Autodesk Fusion 360 part; units mm, degrees
note: some values were not read from the file. Set by a fixed rule: the direction of a hole.
(part 2 of 6)
sketch "Sketch2" plane through (0, 0, 2) normal (0, 0, 1) x (-1, 0, 0)
  line L0 (-25, -25) -> (-154, -25)
  line L1 (-154, -25) -> (-154, -111)
  line L2 (-154, -111) -> (-25, -111)
  line L3 (-25, -111) -> (-25, -25)
  spline S0 degree 3 poles (-57.3506, -87.5946) (-57.8745, -87.5946) (-58.3983, -87.5946) (-58.9381, -87.5946) knots 0 0 0 0 1 1 1 1
  spline S1 degree 3 poles (-58.9381, -87.5946) (-58.9624, -85.5487) (-58.8869, -83.5156) (-58.7793, -81.4728) knots 0 0 0 0 1 1 1 1
  spline S2 degree 3 poles (-58.7793, -81.4728) (-58.764, -81.1715) (-58.7487, -80.8702) (-58.7335, -80.5689) knots 0 0 0 0 1 1 1 1
  spline S3 degree 3 poles (-58.7335, -80.5689) (-58.6965, -79.8416) (-58.6588, -79.1143) (-58.6206, -78.3871) knots 0 0 0 0 1 1 1 1
  spline S4 degree 3 poles (-58.6206, -78.3871) (-58.3587, -78.3871) (-58.0967, -78.3871) (-57.8268, -78.3871) knots 0 0 0 0 1 1 1 1
  spline S5 degree 3 poles (-57.8268, -78.3871) (-57.6309, -79.1758) (-57.6136, -79.9701) (-57.5788, -80.7782) knots 0 0 0 0 1 1 1 1
  spline S6 degree 3 poles (-57.5788, -80.7782) (-57.5721, -80.9263) (-57.5653, -81.0744) (-57.5584, -81.227) knots 0 0 0 0 1 1 1 1
  spline S7 degree 3 poles (-57.5584, -81.227) (-57.5124, -82.2924) (-57.4938, -83.3532) (-57.5093, -84.4196) knots 0 0 0 0 1 1 1 1
  spline S8 degree 3 poles (-57.5093, -84.4196) (-55.2128, -84.0888) (-53.0605, -83.6004) (-50.8806, -82.8013) knots 0 0 0 0 1 1 1 1
  spline S9 degree 3 poles (-50.8806, -82.8013) (-50.4467, -82.6454) (-50.0096, -82.5004) (-49.5718, -82.3558) knots 0 0 0 0 1 1 1 1
  spline S10 degree 3 poles (-49.5718, -82.3558) (-51.0894, -79.4889) (-52.6118, -76.6254) (-54.1756, -73.7833) knots 0 0 0 0 1 1 1 1
  spline S11 degree 3 poles (-54.1756, -73.7833) (-54.0184, -73.6262) (-53.8613, -73.469) (-53.6993, -73.3071) knots 0 0 0 0 1 1 1 1
  spline S12 degree 3 poles (-53.6993, -73.3071) (-53.1237, -73.4989) (-53.084, -73.6261) (-52.7921, -74.1393) knots 0 0 0 0 1 1 1 1
  spline S13 degree 3 poles (-52.7921, -74.1393) (-52.6693, -74.3518) (-52.6693, -74.3518) (-52.5441, -74.5686) knots 0 0 0 0 1 1 1 1
  spline S14 degree 3 poles (-52.5441, -74.5686) (-52.4571, -74.722) (-52.3701, -74.8754) (-52.2805, -75.0335) knots 0 0 0 0 1 1 1 1
  spline S15 degree 3 poles (-52.2805, -75.0335) (-52.0957, -75.353) (-51.9105, -75.6724) (-51.7249, -75.9916) knots 0 0 0 0 1 1 1 1
  spline S16 degree 3 poles (-51.7249, -75.9916) (-51.631, -76.1532) (-51.537, -76.3149) (-51.4403, -76.4815) knots 0 0 0 0 1 1 1 1
  spline S17 degree 3 poles (-51.4403, -76.4815) (-51.0199, -77.195) (-50.5812, -77.8963) (-50.1374, -78.5954) knots 0 0 0 0 1 1 1 1
  spline S18 degree 3 poles (-50.1374, -78.5954) (-50.0252, -78.7727) (-50.0252, -78.7727) (-49.9108, -78.9535) knots 0 0 0 0 1 1 1 1
  spline S19 degree 3 poles (-49.9108, -78.9535) (-49.3861, -79.7779) (-48.8466, -80.592) (-48.3018, -81.4033) knots 0 0 0 0 1 1 1 1
  spline S20 degree 3 poles (-48.3018, -81.4033) (-47.1239, -80.6157) (-46.0109, -79.8094) (-45.0078, -78.8038) knots 0 0 0 0 1 1 1 1
  spline S21 degree 3 poles (-45.0078, -78.8038) (-44.9283, -78.7245) (-44.8489, -78.6453) (-44.767, -78.5636) knots 0 0 0 0 1 1 1 1
  spline S22 degree 3 poles (-44.767, -78.5636) (-44.3785, -78.1633) (-44.0684, -77.795) (-43.8568, -77.2758) knots 0 0 0 0 1 1 1 1
  spline S23 degree 3 poles (-43.8568, -77.2758) (-45.1932, -76.2876) (-46.5379, -75.3133) (-47.8979, -74.3579) knots 0 0 0 0 1 1 1 1
  spline S24 degree 3 poles (-47.8979, -74.3579) (-48.8336, -73.6998) (-49.7613, -73.031) (-50.686, -72.3575) knots 0 0 0 0 1 1 1 1
  spline S25 degree 3 poles (-50.686, -72.3575) (-51.3445, -71.8797) (-52.0085, -71.4118) (-52.6805, -70.9531) knots 0 0 0 0 1 1 1 1
  spline S26 degree 3 poles (-52.6805, -70.9531) (-52.8271, -70.8525) (-52.9738, -70.7519) (-53.1249, -70.6482) knots 0 0 0 0 1 1 1 1
  spline S27 degree 3 poles (-53.1249, -70.6482) (-53.4109, -70.4526) (-53.6978, -70.2583) (-53.9857, -70.0655) knots 0 0 0 0 1 1 1 1
  spline S28 degree 3 poles (-53.9857, -70.0655) (-54.1143, -69.9774) (-54.2428, -69.8892) (-54.3753, -69.7984) knots 0 0 0 0 1 1 1 1
  spline S29 degree 3 poles (-54.3753, -69.7984) (-54.5475, -69.6822) (-54.5475, -69.6822) (-54.7232, -69.5636) knots 0 0 0 0 1 1 1 1
  spline S30 degree 3 poles (-54.7232, -69.5636) (-54.8044, -69.4893) (-54.8857, -69.4149) (-54.9693, -69.3383) knots 0 0 0 0 1 1 1 1
  spline S31 degree 3 poles (-54.9693, -69.3383) (-54.9693, -68.8621) (-54.9693, -68.8621) (-54.8106, -68.5446) knots 0 0 0 0 1 1 1 1
  spline S32 degree 3 poles (-54.8106, -68.5446) (-54.2842, -68.6454) (-53.922, -68.8386) (-53.4767, -69.1337) knots 0 0 0 0 1 1 1 1
  spline S33 degree 3 poles (-53.4767, -69.1337) (-53.3377, -69.2251) (-53.1987, -69.3165) (-53.0555, -69.4107) knots 0 0 0 0 1 1 1 1
  spline S34 degree 3 poles (-53.0555, -69.4107) (-52.829, -69.5615) (-52.829, -69.5615) (-52.598, -69.7153) knots 0 0 0 0 1 1 1 1
  spline S35 degree 3 poles (-52.598, -69.7153) (-52.2685, -69.9326) (-51.939, -70.1499) (-51.6095, -70.3671) knots 0 0 0 0 1 1 1 1
  spline S36 degree 3 poles (-51.6095, -70.3671) (-51.4323, -70.4844) (-51.2551, -70.6016) (-51.0779, -70.7189) knots 0 0 0 0 1 1 1 1
  spline S37 degree 3 poles (-51.0779, -70.7189) (-50.5065, -71.0968) (-49.9333, -71.472) (-49.3598, -71.8467) knots 0 0 0 0 1 1 1 1
  spline S38 degree 3 poles (-49.3598, -71.8467) (-49.162, -71.9759) (-48.9642, -72.1052) (-48.7665, -72.2345) knots 0 0 0 0 1 1 1 1
  spline S39 degree 3 poles (-48.7665, -72.2345) (-48.6684, -72.2985) (-48.5704, -72.3626) (-48.4694, -72.4286) knots 0 0 0 0 1 1 1 1
  spline S40 degree 3 poles (-48.4694, -72.4286) (-46.1202, -73.9643) (-46.1202, -73.9643) (-45.0041, -74.716) knots 0 0 0 0 1 1 1 1
  spline S41 degree 3 poles (-45.0041, -74.716) (-44.8702, -74.8061) (-44.7363, -74.8962) (-44.5984, -74.989) knots 0 0 0 0 1 1 1 1
  spline S42 degree 3 poles (-44.5984, -74.989) (-44.356, -75.1526) (-44.1141, -75.3169) (-43.8728, -75.4819) knots 0 0 0 0 1 1 1 1
  spline S43 degree 3 poles (-43.8728, -75.4819) (-43.3554, -75.8717) (-43.3554, -75.8717) (-42.7456, -76.0058) knots 0 0 0 0 1 1 1 1
  spline S44 degree 3 poles (-42.7456, -76.0058) (-42.2217, -75.0105) (-41.6978, -74.0151) (-41.1581, -72.9896) knots 0 0 0 0 1 1 1 1
  spline S45 degree 3 poles (-41.1581, -72.9896) (-41.6296, -72.8324) (-42.1011, -72.6752) (-42.5868, -72.5133) knots 0 0 0 0 1 1 1 1
  spline S46 degree 3 poles (-42.5868, -72.5133) (-42.8781, -72.3992) (-43.168, -72.2814) (-43.4555, -72.1583) knots 0 0 0 0 1 1 1 1
  spline S47 degree 3 poles (-43.4555, -72.1583) (-43.6096, -72.0926) (-43.7637, -72.0269) (-43.9225, -71.9592) knots 0 0 0 0 1 1 1 1
  spline S48 degree 3 poles (-43.9225, -71.9592) (-44.1644, -71.855) (-44.1644, -71.855) (-44.4112, -71.7487) knots 0 0 0 0 1 1 1 1
  spline S49 degree 3 poles (-44.4112, -71.7487) (-44.5807, -71.6761) (-44.7502, -71.6036) (-44.9249, -71.5288) knots 0 0 0 0 1 1 1 1
  spline S50 degree 3 poles (-44.9249, -71.5288) (-45.2807, -71.3763) (-45.6363, -71.2235) (-45.9919, -71.0705) knots 0 0 0 0 1 1 1 1
  spline S51 degree 3 poles (-45.9919, -71.0705) (-46.5371, -70.836) (-47.0827, -70.6025) (-47.6284, -70.3693) knots 0 0 0 0 1 1 1 1
  spline S52 degree 3 poles (-47.6284, -70.3693) (-47.9749, -70.2206) (-48.3213, -70.0719) (-48.6677, -69.9231) knots 0 0 0 0 1 1 1 1
  spline S53 degree 3 poles (-48.6677, -69.9231) (-48.8309, -69.8533) (-48.9941, -69.7835) (-49.1623, -69.7116) knots 0 0 0 0 1 1 1 1
  spline S54 degree 3 poles (-49.1623, -69.7116) (-49.3134, -69.6464) (-49.4645, -69.5812) (-49.6201, -69.5141) knots 0 0 0 0 1 1 1 1
  spline S55 degree 3 poles (-49.6201, -69.5141) (-49.753, -69.457) (-49.8858, -69.3999) (-50.0226, -69.3411) knots 0 0 0 0 1 1 1 1
  spline S56 degree 3 poles (-50.0226, -69.3411) (-50.3656, -69.1796) (-50.3656, -69.1796) (-50.8418, -68.8621) knots 0 0 0 0 1 1 1 1
  spline S57 degree 3 poles (-50.8418, -68.8621) (-50.7633, -68.5477) (-50.7633, -68.5477) (-50.6831, -68.2271) knots 0 0 0 0 1 1 1 1
  spline S58 degree 3 poles (-50.6831, -68.2271) (-49.5395, -68.587) (-48.4525, -69.0329) (-47.3549, -69.5138) knots 0 0 0 0 1 1 1 1
  spline S59 degree 3 poles (-47.3549, -69.5138) (-47.178, -69.5907) (-47.0011, -69.6675) (-46.8188, -69.7467) knots 0 0 0 0 1 1 1 1
  spline S60 degree 3 poles (-46.8188, -69.7467) (-46.2578, -69.9903) (-45.6973, -70.2347) (-45.1368, -70.4793) knots 0 0 0 0 1 1 1 1
  spline S61 degree 3 poles (-45.1368, -70.4793) (-44.3948, -70.8031) (-43.6524, -71.126) (-42.9099, -71.4486) knots 0 0 0 0 1 1 1 1
  spline S62 degree 3 poles (-42.9099, -71.4486) (-42.7389, -71.5235) (-42.568, -71.5984) (-42.3918, -71.6755) knots 0 0 0 0 1 1 1 1
  spline S63 degree 3 poles (-42.3918, -71.6755) (-42.2344, -71.7439) (-42.0769, -71.8123) (-41.9147, -71.8828) knots 0 0 0 0 1 1 1 1
  spline S64 degree 3 poles (-41.9147, -71.8828) (-41.7759, -71.9434) (-41.637, -72.004) (-41.494, -72.0664) knots 0 0 0 0 1 1 1 1
  spline S65 degree 3 poles (-41.494, -72.0664) (-41.1687, -72.2148) (-41.1687, -72.2148) (-40.8406, -72.1958) knots 0 0 0 0 1 1 1 1
  spline S66 degree 3 poles (-40.8406, -72.1958) (-40.5787, -71.3576) (-40.3167, -70.5194) (-40.0468, -69.6558) knots 0 0 0 0 1 1 1 1
  spline S67 degree 3 poles (-40.0468, -69.6558) (-40.425, -69.5969) (-40.425, -69.5969) (-40.8108, -69.5368) knots 0 0 0 0 1 1 1 1
  spline S68 degree 3 poles (-40.8108, -69.5368) (-41.7318, -69.3834) (-42.6454, -69.2019) (-43.5592, -69.0109) knots 0 0 0 0 1 1 1 1
  spline S69 degree 3 poles (-43.5592, -69.0109) (-43.7596, -68.9694) (-43.7596, -68.9694) (-43.964, -68.927) knots 0 0 0 0 1 1 1 1
  spline S70 degree 3 poles (-43.964, -68.927) (-44.0895, -68.9005) (-44.215, -68.8739) (-44.3443, -68.8466) knots 0 0 0 0 1 1 1 1
  spline S71 degree 3 poles (-44.3443, -68.8466) (-44.4568, -68.8228) (-44.5694, -68.7991) (-44.6854, -68.7746) knots 0 0 0 0 1 1 1 1
  spline S72 degree 3 poles (-44.6854, -68.7746) (-44.9681, -68.7033) (-44.9681, -68.7033) (-45.2856, -68.5446) knots 0 0 0 0 1 1 1 1
  spline S73 degree 3 poles (-45.2856, -68.5446) (-45.2332, -68.2826) (-45.1808, -68.0207) (-45.1268, -67.7508) knots 0 0 0 0 1 1 1 1
  spline S74 degree 3 poles (-45.1268, -67.7508) (-44.4572, -67.8377) (-43.7877, -67.9253) (-43.1182, -68.0134) knots 0 0 0 0 1 1 1 1
  spline S75 degree 3 poles (-43.1182, -68.0134) (-42.8905, -68.0433) (-42.6628, -68.073) (-42.435, -68.1025) knots 0 0 0 0 1 1 1 1
  spline S76 degree 3 poles (-42.435, -68.1025) (-42.1075, -68.1451) (-41.7801, -68.1882) (-41.4526, -68.2314) knots 0 0 0 0 1 1 1 1
  spline S77 degree 3 poles (-41.4526, -68.2314) (-41.1571, -68.2701) (-41.1571, -68.2701) (-40.8556, -68.3095) knots 0 0 0 0 1 1 1 1
  spline S78 degree 3 poles (-40.8556, -68.3095) (-40.3643, -68.3858) (-40.3643, -68.3858) (-39.8881, -68.5446) knots 0 0 0 0 1 1 1 1
  spline S79 degree 3 poles (-39.8881, -68.5446) (-39.8357, -67.7588) (-39.7833, -66.9729) (-39.7293, -66.1633) knots 0 0 0 0 1 1 1 1
  spline S80 degree 3 poles (-39.7293, -66.1633) (-40.9343, -66.1633) (-42.1392, -66.1633) (-43.3806, -66.1633) knots 0 0 0 0 1 1 1 1
  spline S81 degree 3 poles (-43.3806, -66.1633) (-43.3806, -65.9538) (-43.3806, -65.7442) (-43.3806, -65.5283) knots 0 0 0 0 1 1 1 1
  spline S82 degree 3 poles (-43.3806, -65.5283) (-41.9137, -65.5283) (-40.4469, -65.5283) (-38.9356, -65.5283) knots 0 0 0 0 1 1 1 1
  spline S83 degree 3 poles (-38.9356, -65.5283) (-38.9356, -66.6399) (-38.9521, -67.6188) (-39.0943, -68.7033) knots 0 0 0 0 1 1 1 1
  spline S84 degree 3 poles (-39.0943, -68.7033) (-38.9726, -68.711) (-38.8509, -68.7186) (-38.7256, -68.7265) knots 0 0 0 0 1 1 1 1
  spline S85 degree 3 poles (-38.7256, -68.7265) (-37.3659, -68.8206) (-36.0268, -68.9891) (-34.6791, -69.1895) knots 0 0 0 0 1 1 1 1
  spline S86 degree 3 poles (-34.6791, -69.1895) (-34.4764, -69.2191) (-34.2737, -69.2486) (-34.0649, -69.2791) knots 0 0 0 0 1 1 1 1
  spline S87 degree 3 poles (-34.0649, -69.2791) (-33.5717, -69.3511) (-33.0786, -69.4238) (-32.5856, -69.4971) knots 0 0 0 0 1 1 1 1
  spline S88 degree 3 poles (-32.5856, -69.4971) (-32.638, -70.0733) (-32.6904, -70.6496) (-32.7443, -71.2433) knots 0 0 0 0 1 1 1 1
  spline S89 degree 3 poles (-32.7443, -71.2433) (-33.6174, -71.0657) (-34.4904, -70.8878) (-35.3634, -70.7094) knots 0 0 0 0 1 1 1 1
  spline S90 degree 3 poles (-35.3634, -70.7094) (-35.6604, -70.6488) (-35.9574, -70.5883) (-36.2545, -70.5279) knots 0 0 0 0 1 1 1 1
  spline S91 degree 3 poles (-36.2545, -70.5279) (-36.6813, -70.4411) (-37.108, -70.3539) (-37.5347, -70.2666) knots 0 0 0 0 1 1 1 1
  spline S92 degree 3 poles (-37.5347, -70.2666) (-37.6677, -70.2397) (-37.8007, -70.2127) (-37.9377, -70.1849) knots 0 0 0 0 1 1 1 1
  spline S93 degree 3 poles (-37.9377, -70.1849) (-38.0616, -70.1595) (-38.1855, -70.1341) (-38.3132, -70.1079) knots 0 0 0 0 1 1 1 1
  spline S94 degree 3 poles (-38.3132, -70.1079) (-38.4221, -70.0857) (-38.531, -70.0635) (-38.6433, -70.0406) knots 0 0 0 0 1 1 1 1
  spline S95 degree 3 poles (-38.6433, -70.0406) (-38.9356, -69.9733) (-38.9356, -69.9733) (-39.4118, -69.8146) knots 0 0 0 0 1 1 1 1
  spline S96 degree 3 poles (-39.4118, -69.8146) (-39.428, -69.9942) (-39.4442, -70.1739) (-39.4608, -70.359) knots 0 0 0 0 1 1 1 1
  spline S97 degree 3 poles (-39.4608, -70.359) (-39.5577, -71.1252) (-39.7863, -71.8123) (-40.0568, -72.5332) knots 0 0 0 0 1 1 1 1
  spline S98 degree 3 poles (-40.0568, -72.5332) (-40.1051, -72.6637) (-40.1534, -72.7943) (-40.2032, -72.9288) knots 0 0 0 0 1 1 1 1
  spline S99 degree 3 poles (-40.2032, -72.9288) (-40.6069, -73.982) (-41.1105, -74.9355) (-41.6976, -75.8967) knots 0 0 0 0 1 1 1 1
  spline S100 degree 3 poles (-41.6976, -75.8967) (-41.9685, -76.3167) (-41.9685, -76.3167) (-42.1106, -76.7996) knots 0 0 0 0 1 1 1 1
  spline S101 degree 3 poles (-42.1106, -76.7996) (-42.0027, -76.837) (-41.8948, -76.8744) (-41.7837, -76.913) knots 0 0 0 0 1 1 1 1
  spline S102 degree 3 poles (-41.7837, -76.913) (-41.2117, -77.163) (-40.7122, -77.4938) (-40.1975, -77.8426) knots 0 0 0 0 1 1 1 1
  spline S103 degree 3 poles (-40.1975, -77.8426) (-40.0929, -77.9126) (-39.9884, -77.9826) (-39.8806, -78.0548) knots 0 0 0 0 1 1 1 1
  spline S104 degree 3 poles (-39.8806, -78.0548) (-39.5486, -78.2773) (-39.2173, -78.5008) (-38.886, -78.7244) knots 0 0 0 0 1 1 1 1
  spline S105 degree 3 poles (-38.886, -78.7244) (-38.6602, -78.876) (-38.4344, -79.0275) (-38.2085, -79.179) knots 0 0 0 0 1 1 1 1
  spline S106 degree 3 poles (-38.2085, -79.179) (-37.6566, -79.5492) (-37.1053, -79.9204) (-36.5543, -80.2921) knots 0 0 0 0 1 1 1 1
  spline S107 degree 3 poles (-36.5543, -80.2921) (-37.0937, -81.3516) (-37.0937, -81.3516) (-37.5085, -81.5759) knots 0 0 0 0 1 1 1 1
  spline S108 degree 3 poles (-37.5085, -81.5759) (-37.9253, -81.5576) (-38.101, -81.4328) (-38.4333, -81.1819) knots 0 0 0 0 1 1 1 1
  spline S109 degree 3 poles (-38.4333, -81.1819) (-38.5489, -81.0963) (-38.6646, -81.0107) (-38.7837, -80.9225) knots 0 0 0 0 1 1 1 1
  spline S110 degree 3 poles (-38.7837, -80.9225) (-38.9059, -80.8291) (-39.028, -80.7356) (-39.1539, -80.6393) knots 0 0 0 0 1 1 1 1
  spline S111 degree 3 poles (-39.1539, -80.6393) (-39.4093, -80.4491) (-39.6648, -80.2589) (-39.9203, -80.0688) knots 0 0 0 0 1 1 1 1
  spline S112 degree 3 poles (-39.9203, -80.0688) (-40.0477, -79.9731) (-40.1751, -79.8773) (-40.3064, -79.7786) knots 0 0 0 0 1 1 1 1
  spline S113 degree 3 poles (-40.3064, -79.7786) (-40.8553, -79.3688) (-41.4129, -78.9718) (-41.9717, -78.5756) knots 0 0 0 0 1 1 1 1
  spline S114 degree 3 poles (-41.9717, -78.5756) (-42.154, -78.4456) (-42.3363, -78.3156) (-42.5186, -78.1855) knots 0 0 0 0 1 1 1 1
  spline S115 degree 3 poles (-42.5186, -78.1855) (-42.6459, -78.0949) (-42.7732, -78.0042) (-42.9043, -77.9108) knots 0 0 0 0 1 1 1 1
  spline S116 degree 3 poles (-42.9043, -77.9108) (-43.0212, -78.0277) (-43.138, -78.1445) (-43.2584, -78.2649) knots 0 0 0 0 1 1 1 1
  spline S117 degree 3 poles (-43.2584, -78.2649) (-43.8283, -78.8348) (-44.3982, -79.4047) (-44.9681, -79.9746) knots 0 0 0 0 1 1 1 1
  spline S118 degree 3 poles (-44.9681, -79.9746) (-44.2568, -80.8305) (-43.4993, -81.6123) (-42.7016, -82.3874) knots 0 0 0 0 1 1 1 1
  spline S119 degree 3 poles (-42.7016, -82.3874) (-42.4506, -82.634) (-42.1998, -82.8808) (-41.949, -83.1276) knots 0 0 0 0 1 1 1 1
  spline S120 degree 3 poles (-41.949, -83.1276) (-41.5566, -83.5131) (-41.1636, -83.898) (-40.7689, -84.2813) knots 0 0 0 0 1 1 1 1
  spline S121 degree 3 poles (-40.7689, -84.2813) (-40.3861, -84.6537) (-40.0058, -85.0284) (-39.6258, -85.4037) knots 0 0 0 0 1 1 1 1
  spline S122 degree 3 poles (-39.6258, -85.4037) (-39.5064, -85.5185) (-39.387, -85.6332) (-39.2641, -85.7515) knots 0 0 0 0 1 1 1 1
  spline S123 degree 3 poles (-39.2641, -85.7515) (-39.1559, -85.8591) (-39.0477, -85.9667) (-38.9362, -86.0776) knots 0 0 0 0 1 1 1 1
  spline S124 degree 3 poles (-38.9362, -86.0776) (-38.8401, -86.1715) (-38.7439, -86.2655) (-38.6448, -86.3622) knots 0 0 0 0 1 1 1 1
  spline S125 degree 3 poles (-38.6448, -86.3622) (-38.4593, -86.6421) (-38.4593, -86.6421) (-38.5089, -86.9948) knots 0 0 0 0 1 1 1 1
  spline S126 degree 3 poles (-38.5089, -86.9948) (-38.5449, -87.088) (-38.581, -87.1811) (-38.6181, -87.2771) knots 0 0 0 0 1 1 1 1
  spline S127 degree 3 poles (-38.6181, -87.2771) (-39.0954, -87.0643) (-39.4115, -86.8328) (-39.769, -86.4535) knots 0 0 0 0 1 1 1 1
  spline S128 degree 3 poles (-39.769, -86.4535) (-40.1306, -86.0714) (-40.5076, -85.7239) (-40.9076, -85.3832) knots 0 0 0 0 1 1 1 1
  spline S129 degree 3 poles (-40.9076, -85.3832) (-41.8861, -84.5338) (-42.7858, -83.6024) (-43.6981, -82.6832) knots 0 0 0 0 1 1 1 1
  spline S130 degree 3 poles (-43.6981, -82.6832) (-43.8835, -82.4971) (-44.0689, -82.3109) (-44.2543, -82.1248) knots 0 0 0 0 1 1 1 1
  spline S131 degree 3 poles (-44.2543, -82.1248) (-44.7043, -81.6731) (-45.1539, -81.2208) (-45.6031, -80.7683) knots 0 0 0 0 1 1 1 1
  spline S132 degree 3 poles (-45.6031, -80.7683) (-46.1303, -81.0241) (-46.5933, -81.3215) (-47.0715, -81.6613) knots 0 0 0 0 1 1 1 1
  spline S133 degree 3 poles (-47.0715, -81.6613) (-47.2131, -81.7616) (-47.3547, -81.8618) (-47.5006, -81.9651) knots 0 0 0 0 1 1 1 1
  spline S134 degree 3 poles (-47.5006, -81.9651) (-47.6079, -82.0417) (-47.7151, -82.1182) (-47.8256, -82.1971) knots 0 0 0 0 1 1 1 1
  spline S135 degree 3 poles (-47.8256, -82.1971) (-47.6276, -82.5479) (-47.4291, -82.8984) (-47.2303, -83.2488) knots 0 0 0 0 1 1 1 1
  spline S136 degree 3 poles (-47.2303, -83.2488) (-47.175, -83.3468) (-47.1198, -83.4448) (-47.0628, -83.5458) knots 0 0 0 0 1 1 1 1
  spline S137 degree 3 poles (-47.0628, -83.5458) (-46.79, -84.0258) (-46.5106, -84.4926) (-46.1972, -84.9473) knots 0 0 0 0 1 1 1 1
  spline S138 degree 3 poles (-46.1972, -84.9473) (-45.9206, -85.3721) (-45.9206, -85.3721) (-45.9007, -85.7193) knots 0 0 0 0 1 1 1 1
  spline S139 degree 3 poles (-45.9007, -85.7193) (-46.1781, -86.1661) (-46.5558, -86.289) (-47.0318, -86.4833) knots 0 0 0 0 1 1 1 1
  spline S140 degree 3 poles (-47.0318, -86.4833) (-47.1366, -86.4833) (-47.2414, -86.4833) (-47.3493, -86.4833) knots 0 0 0 0 1 1 1 1
  spline S141 degree 3 poles (-47.3493, -86.4833) (-47.9256, -85.3832) (-48.5019, -84.283) (-49.0956, -83.1496) knots 0 0 0 0 1 1 1 1
  spline S142 degree 3 poles (-49.0956, -83.1496) (-49.795, -83.2894) (-50.3211, -83.4767) (-50.9708, -83.7548) knots 0 0 0 0 1 1 1 1
  spline S143 degree 3 poles (-50.9708, -83.7548) (-52.8284, -84.524) (-54.8494, -85.0961) (-56.8743, -85.0645) knots 0 0 0 0 1 1 1 1
  spline S144 degree 3 poles (-56.8743, -85.0645) (-56.9955, -85.0631) (-57.1166, -85.0616) (-57.2414, -85.0601) knots 0 0 0 0 1 1 1 1
  spline S145 degree 3 poles (-57.2414, -85.0601) (-57.3299, -85.0583) (-57.4183, -85.0565) (-57.5093, -85.0546) knots 0 0 0 0 1 1 1 1
  spline S146 degree 3 poles (-57.5093, -85.0546) (-57.4831, -85.179) (-57.457, -85.3034) (-57.43, -85.4316) knots 0 0 0 0 1 1 1 1
  spline S147 degree 3 poles (-57.43, -85.4316) (-57.3294, -86.1605) (-57.3406, -86.8588) (-57.3506, -87.5946) knots 0 0 0 0 1 1 1 1
  spline S148 degree 3 poles (-68.1456, -65.8458) (-68.3551, -65.7934) (-68.5647, -65.741) (-68.7806, -65.6871) knots 0 0 0 0 1 1 1 1
  spline S149 degree 3 poles (-68.7806, -65.6871) (-68.7806, -65.3204) (-68.7806, -64.9536) (-68.7806, -64.5758) knots 0 0 0 0 1 1 1 1
  spline S150 degree 3 poles (-68.7806, -64.5758) (-68.8977, -64.5691) (-69.0148, -64.5623) (-69.1354, -64.5554) knots 0 0 0 0 1 1 1 1
  spline S151 degree 3 poles (-69.1354, -64.5554) (-70.6364, -64.4558) (-72.1077, -64.2436) (-73.5927, -64.0103) knots 0 0 0 0 1 1 1 1
  spline S152 degree 3 poles (-73.5927, -64.0103) (-73.8357, -63.9727) (-74.0787, -63.9352) (-74.3216, -63.8977) knots 0 0 0 0 1 1 1 1
  spline S153 degree 3 poles (-74.3216, -63.8977) (-74.9089, -63.8071) (-75.496, -63.7155) (-76.0831, -63.6233) knots 0 0 0 0 1 1 1 1
  spline S154 degree 3 poles (-76.0831, -63.6233) (-76.0307, -63.0994) (-75.9783, -62.5756) (-75.9243, -62.0358) knots 0 0 0 0 1 1 1 1
  spline S155 degree 3 poles (-75.9243, -62.0358) (-74.5265, -62.1244) (-73.1989, -62.3743) (-71.8343, -62.6726) knots 0 0 0 0 1 1 1 1
  spline S156 degree 3 poles (-71.8343, -62.6726) (-71.4758, -62.751) (-71.117, -62.8279) (-70.7581, -62.9046) knots 0 0 0 0 1 1 1 1
  spline S157 degree 3 poles (-70.7581, -62.9046) (-70.5289, -62.9539) (-70.2997, -63.0033) (-70.0704, -63.0528) knots 0 0 0 0 1 1 1 1
  spline S158 degree 3 poles (-70.0704, -63.0528) (-69.9105, -63.0873) (-69.9105, -63.0873) (-69.7472, -63.1225) knots 0 0 0 0 1 1 1 1
  spline S159 degree 3 poles (-69.7472, -63.1225) (-69.3095, -63.2183) (-68.8887, -63.3227) (-68.4631, -63.4646) knots 0 0 0 0 1 1 1 1
  spline S160 degree 3 poles (-68.4631, -63.4646) (-68.4438, -63.2334) (-68.4438, -63.2334) (-68.424, -62.9976) knots 0 0 0 0 1 1 1 1
  spline S161 degree 3 poles (-68.424, -62.9976) (-68.3162, -62.243) (-67.9954, -61.6117) (-67.6594, -60.9345) knots 0 0 0 0 1 1 1 1
  spline S162 degree 3 poles (-67.6594, -60.9345) (-67.5996, -60.8108) (-67.5397, -60.6871) (-67.478, -60.5596) knots 0 0 0 0 1 1 1 1
  spline S163 degree 3 poles (-67.478, -60.5596) (-67.3315, -60.2573) (-67.1831, -59.9558) (-67.0343, -59.6546) knots 0 0 0 0 1 1 1 1
  spline S164 degree 3 poles (-67.0343, -59.6546) (-67.1091, -59.5997) (-67.1838, -59.5449) (-67.2608, -59.4883) knots 0 0 0 0 1 1 1 1
  spline S165 degree 3 poles (-67.2608, -59.4883) (-68.7252, -58.413) (-70.186, -57.3333) (-71.6381, -56.2414) knots 0 0 0 0 1 1 1 1
  spline S166 degree 3 poles (-71.6381, -56.2414) (-72.6697, -55.4659) (-73.7042, -54.6947) (-74.7436, -53.9296) knots 0 0 0 0 1 1 1 1
  spline S167 degree 3 poles (-74.7436, -53.9296) (-74.8656, -53.8398) (-74.9876, -53.75) (-75.1132, -53.6575) knots 0 0 0 0 1 1 1 1
  spline S168 degree 3 poles (-75.1132, -53.6575) (-75.7696, -53.1747) (-76.4268, -52.6929) (-77.0846, -52.2119) knots 0 0 0 0 1 1 1 1
  spline S169 degree 3 poles (-77.0846, -52.2119) (-77.2225, -52.1108) (-77.3604, -52.0098) (-77.5025, -51.9056) knots 0 0 0 0 1 1 1 1
  spline S170 degree 3 poles (-77.5025, -51.9056) (-77.7672, -51.7117) (-78.0321, -51.518) (-78.2973, -51.3248) knots 0 0 0 0 1 1 1 1
  spline S171 degree 3 poles (-78.2973, -51.3248) (-78.4162, -51.2375) (-78.5352, -51.1503) (-78.6578, -51.0604) knots 0 0 0 0 1 1 1 1
  spline S172 degree 3 poles (-78.6578, -51.0604) (-78.8148, -50.9457) (-78.8148, -50.9457) (-78.975, -50.8286) knots 0 0 0 0 1 1 1 1
  spline S173 degree 3 poles (-78.975, -50.8286) (-79.2581, -50.6058) (-79.2581, -50.6058) (-79.7343, -50.1296) knots 0 0 0 0 1 1 1 1
  spline S174 degree 3 poles (-79.7343, -50.1296) (-79.42, -49.7105) (-79.1057, -49.2914) (-78.7818, -48.8596) knots 0 0 0 0 1 1 1 1
  spline S175 degree 3 poles (-78.7818, -48.8596) (-78.0892, -49.3033) (-77.4591, -49.7891) (-76.8372, -50.328) knots 0 0 0 0 1 1 1 1
  spline S176 degree 3 poles (-76.8372, -50.328) (-76.223, -50.8542) (-75.6063, -51.374) (-74.9718, -51.8758) knots 0 0 0 0 1 1 1 1
  spline S177 degree 3 poles (-74.9718, -51.8758) (-74.2607, -52.4391) (-73.5695, -53.0235) (-72.8789, -53.6115) knots 0 0 0 0 1 1 1 1
  spline S178 degree 3 poles (-72.8789, -53.6115) (-72.3661, -54.0472) (-71.8481, -54.4742) (-71.3206, -54.8921) knots 0 0 0 0 1 1 1 1
  spline S179 degree 3 poles (-71.3206, -54.8921) (-70.7012, -55.3827) (-70.0965, -55.8881) (-69.495, -56.4002) knots 0 0 0 0 1 1 1 1
  spline S180 degree 3 poles (-69.495, -56.4002) (-67.971, -57.7848) (-67.971, -57.7848) (-66.2406, -58.8608) knots 0 0 0 0 1 1 1 1
  spline S181 degree 3 poles (-66.2406, -58.8608) (-66.1557, -58.7452) (-66.0707, -58.6296) (-65.9832, -58.5104) knots 0 0 0 0 1 1 1 1
  spline S182 degree 3 poles (-65.9832, -58.5104) (-65.5749, -58.031) (-65.1512, -57.6937) (-64.6432, -57.3229) knots 0 0 0 0 1 1 1 1
  spline S183 degree 3 poles (-64.6432, -57.3229) (-64.4776, -57.2012) (-64.3121, -57.0794) (-64.1415, -56.954) knots 0 0 0 0 1 1 1 1
  spline S184 degree 3 poles (-64.1415, -56.954) (-63.8394, -56.7377) (-63.5334, -56.5269) (-63.2243, -56.3208) knots 0 0 0 0 1 1 1 1
  spline S185 degree 3 poles (-63.2243, -56.3208) (-63.2769, -56.2404) (-63.3294, -56.16) (-63.3836, -56.0772) knots 0 0 0 0 1 1 1 1
  spline S186 degree 3 poles (-63.3836, -56.0772) (-64.386, -54.5424) (-65.3844, -53.005) (-66.3696, -51.4591) knots 0 0 0 0 1 1 1 1
  spline S187 degree 3 poles (-66.3696, -51.4591) (-66.4523, -51.3304) (-66.535, -51.2017) (-66.6203, -51.0692) knots 0 0 0 0 1 1 1 1
  spline S188 degree 3 poles (-66.6203, -51.0692) (-66.6957, -50.9502) (-66.7712, -50.8313) (-66.8489, -50.7088) knots 0 0 0 0 1 1 1 1
  spline S189 degree 3 poles (-66.8489, -50.7088) (-66.9156, -50.6043) (-66.9823, -50.4998) (-67.051, -50.3921) knots 0 0 0 0 1 1 1 1
  spline S190 degree 3 poles (-67.051, -50.3921) (-67.1931, -50.1296) (-67.1931, -50.1296) (-67.1931, -49.8121) knots 0 0 0 0 1 1 1 1
  spline S191 degree 3 poles (-67.1931, -49.8121) (-66.3714, -49.3005) (-66.3714, -49.3005) (-66.0818, -49.1771) knots 0 0 0 0 1 1 1 1
  spline S192 degree 3 poles (-66.0818, -49.1771) (-65.427, -49.3953) (-65.3789, -49.6875) (-65.0717, -50.297) knots 0 0 0 0 1 1 1 1
  spline S193 degree 3 poles (-65.0717, -50.297) (-65.0217, -50.3948) (-64.9718, -50.4926) (-64.9204, -50.5934) knots 0 0 0 0 1 1 1 1
  spline S194 degree 3 poles (-64.9204, -50.5934) (-64.7604, -50.9077) (-64.6025, -51.223) (-64.4447, -51.5385) knots 0 0 0 0 1 1 1 1
  spline S195 degree 3 poles (-64.4447, -51.5385) (-64.2887, -51.847) (-64.1323, -52.1553) (-63.9757, -52.4636) knots 0 0 0 0 1 1 1 1
  spline S196 degree 3 poles (-63.9757, -52.4636) (-63.8732, -52.6656) (-63.771, -52.8677) (-63.669, -53.07) knots 0 0 0 0 1 1 1 1
  spline S197 degree 3 poles (-63.669, -53.07) (-63.2779, -53.8435) (-62.8643, -54.6028) (-62.4373, -55.3572) knots 0 0 0 0 1 1 1 1
  spline S198 degree 3 poles (-62.4373, -55.3572) (-62.2718, -55.6858) (-62.2718, -55.6858) (-62.2718, -56.0033) knots 0 0 0 0 1 1 1 1
  spline S199 degree 3 poles (-62.2718, -56.0033) (-61.8527, -55.8462) (-61.4336, -55.689) (-61.0018, -55.5271) knots 0 0 0 0 1 1 1 1
  spline S200 degree 3 poles (-61.0018, -55.5271) (-61.0259, -55.3886) (-61.0499, -55.2502) (-61.0747, -55.1075) knots 0 0 0 0 1 1 1 1
  spline S201 degree 3 poles (-61.0747, -55.1075) (-61.1642, -54.5896) (-61.2529, -54.0715) (-61.341, -53.5533) knots 0 0 0 0 1 1 1 1
  spline S202 degree 3 poles (-61.341, -53.5533) (-61.3791, -53.3299) (-61.4176, -53.1065) (-61.4565, -52.8832) knots 0 0 0 0 1 1 1 1
  spline S203 degree 3 poles (-61.4565, -52.8832) (-61.5125, -52.5605) (-61.5673, -52.2377) (-61.622, -51.9149) knots 0 0 0 0 1 1 1 1
  spline S204 degree 3 poles (-61.622, -51.9149) (-61.6552, -51.7212) (-61.6885, -51.5275) (-61.7227, -51.3279) knots 0 0 0 0 1 1 1 1
  spline S205 degree 3 poles (-61.7227, -51.3279) (-61.7958, -50.7629) (-61.8084, -50.2223) (-61.7956, -49.6533) knots 0 0 0 0 1 1 1 1
  spline S206 degree 3 poles (-61.7956, -49.6533) (-61.586, -49.6533) (-61.3765, -49.6533) (-61.1606, -49.6533) knots 0 0 0 0 1 1 1 1
  spline S207 degree 3 poles (-61.1606, -49.6533) (-61.0242, -50.365) (-60.8886, -51.0769) (-60.7536, -51.7888) knots 0 0 0 0 1 1 1 1
  spline S208 degree 3 poles (-60.7536, -51.7888) (-60.7076, -52.0309) (-60.6614, -52.273) (-60.615, -52.515) knots 0 0 0 0 1 1 1 1
  spline S209 degree 3 poles (-60.615, -52.515) (-60.5483, -52.8632) (-60.4823, -53.2116) (-60.4164, -53.5601) knots 0 0 0 0 1 1 1 1
  spline S210 degree 3 poles (-60.4164, -53.5601) (-60.3956, -53.6679) (-60.3748, -53.7757) (-60.3533, -53.8868) knots 0 0 0 0 1 1 1 1
  spline S211 degree 3 poles (-60.3533, -53.8868) (-60.2579, -54.3956) (-60.2081, -54.8475) (-60.2081, -55.3683) knots 0 0 0 0 1 1 1 1
  spline S212 degree 3 poles (-60.2081, -55.3683) (-60.0804, -55.3421) (-59.9527, -55.3159) (-59.8211, -55.2889) knots 0 0 0 0 1 1 1 1
  spline S213 degree 3 poles (-59.8211, -55.2889) (-59.151, -55.1949) (-58.5021, -55.1961) (-57.8268, -55.2096) knots 0 0 0 0 1 1 1 1
  spline S214 degree 3 poles (-57.8268, -55.2096) (-57.8268, -55.4715) (-57.8268, -55.7334) (-57.8268, -56.0033) knots 0 0 0 0 1 1 1 1
  spline S215 degree 3 poles (-57.8268, -56.0033) (-57.9556, -56.0092) (-58.0843, -56.0152) (-58.2169, -56.0213) knots 0 0 0 0 1 1 1 1
  spline S216 degree 3 poles (-58.2169, -56.0213) (-59.4131, -56.0923) (-60.4952, -56.2746) (-61.6368, -56.6383) knots 0 0 0 0 1 1 1 1
  spline S217 degree 3 poles (-61.6368, -56.6383) (-61.5845, -56.7824) (-61.5321, -56.9264) (-61.4781, -57.0749) knots 0 0 0 0 1 1 1 1
  spline S218 degree 3 poles (-61.4781, -57.0749) (-61.3193, -57.5908) (-61.3193, -57.5908) (-61.3193, -58.2258) knots 0 0 0 0 1 1 1 1
  spline S219 degree 3 poles (-61.3193, -58.2258) (-61.6337, -58.3044) (-61.6337, -58.3044) (-61.9543, -58.3846) knots 0 0 0 0 1 1 1 1
  spline S220 degree 3 poles (-61.9543, -58.3846) (-62.5893, -57.4718) (-62.5893, -57.4718) (-62.5893, -57.1146) knots 0 0 0 0 1 1 1 1
  spline S221 degree 3 poles (-62.5893, -57.1146) (-63.1132, -57.4289) (-63.6371, -57.7432) (-64.1768, -58.0671) knots 0 0 0 0 1 1 1 1
  spline S222 degree 3 poles (-64.1768, -58.0671) (-63.8906, -58.7826) (-63.7207, -59.0611) (-63.2144, -59.595) knots 0 0 0 0 1 1 1 1
  spline S223 degree 3 poles (-63.2144, -59.595) (-62.6745, -60.1796) (-62.1472, -60.7702) (-61.6368, -61.381) knots 0 0 0 0 1 1 1 1
  spline S224 degree 3 poles (-61.6368, -61.381) (-61.519, -61.5214) (-61.4011, -61.6617) (-61.2797, -61.8064) knots 0 0 0 0 1 1 1 1
  spline S225 degree 3 poles (-61.2797, -61.8064) (-61.0218, -62.1667) (-60.9075, -62.3971) (-60.8431, -62.8296) knots 0 0 0 0 1 1 1 1
  spline S226 degree 3 poles (-60.8431, -62.8296) (-61.0003, -62.9343) (-61.1574, -63.0391) (-61.3193, -63.1471) knots 0 0 0 0 1 1 1 1
  spline S227 degree 3 poles (-61.3193, -63.1471) (-62.3114, -62.0659) (-63.254, -60.9539) (-64.1768, -59.8133) knots 0 0 0 0 1 1 1 1
  spline S228 degree 3 poles (-64.1768, -59.8133) (-64.4402, -59.4947) (-64.7051, -59.1776) (-64.9706, -58.8608) knots 0 0 0 0 1 1 1 1
  spline S229 degree 3 poles (-64.9706, -58.8608) (-65.8193, -59.686) (-66.4563, -60.484) (-66.9748, -61.5496) knots 0 0 0 0 1 1 1 1
  spline S230 degree 3 poles (-66.9748, -61.5496) (-67.0223, -61.6441) (-67.0698, -61.7385) (-67.1187, -61.8358) knots 0 0 0 0 1 1 1 1
  spline S231 degree 3 poles (-67.1187, -61.8358) (-67.4068, -62.4191) (-67.6364, -63.0019) (-67.8281, -63.6233) knots 0 0 0 0 1 1 1 1
  spline S232 degree 3 poles (-67.8281, -63.6233) (-67.7141, -63.6414) (-67.6, -63.6595) (-67.4825, -63.6781) knots 0 0 0 0 1 1 1 1
  spline S233 degree 3 poles (-67.4825, -63.6781) (-66.2806, -63.873) (-65.09, -64.1046) (-63.899, -64.3575) knots 0 0 0 0 1 1 1 1
  spline S234 degree 3 poles (-63.899, -64.3575) (-63.7259, -64.394) (-63.5528, -64.4304) (-63.3744, -64.4679) knots 0 0 0 0 1 1 1 1
  spline S235 degree 3 poles (-63.3744, -64.4679) (-62.9539, -64.5564) (-62.5335, -64.6453) (-62.1131, -64.7346) knots 0 0 0 0 1 1 1 1
  spline S236 degree 3 poles (-62.1131, -64.7346) (-62.1131, -64.9965) (-62.1131, -65.2584) (-62.1131, -65.5283) knots 0 0 0 0 1 1 1 1
  spline S237 degree 3 poles (-62.1131, -65.5283) (-64.1461, -65.4475) (-66.1429, -65.0714) (-68.1456, -64.7346) knots 0 0 0 0 1 1 1 1
  spline S238 degree 3 poles (-68.1456, -64.7346) (-68.1456, -65.1013) (-68.1456, -65.468) (-68.1456, -65.8458) knots 0 0 0 0 1 1 1 1
  spline S239 degree 3 poles (-63.0656, -81.0858) (-63.6419, -81.0858) (-64.2181, -81.0858) (-64.8118, -81.0858) knots 0 0 0 0 1 1 1 1
  spline S240 degree 3 poles (-64.8118, -81.0858) (-65.3455, -79.8056) (-65.7807, -78.5056) (-66.1978, -77.1834) knots 0 0 0 0 1 1 1 1
  spline S241 degree 3 poles (-66.1978, -77.1834) (-66.2677, -76.9633) (-66.3376, -76.7433) (-66.4075, -76.5232) knots 0 0 0 0 1 1 1 1
  spline S242 degree 3 poles (-66.4075, -76.5232) (-66.5529, -76.0653) (-66.6979, -75.6073) (-66.8425, -75.1492) knots 0 0 0 0 1 1 1 1
  spline S243 degree 3 poles (-66.8425, -75.1492) (-67.0276, -74.5632) (-67.2135, -73.9776) (-67.3998, -73.392) knots 0 0 0 0 1 1 1 1
  spline S244 degree 3 poles (-67.3998, -73.392) (-67.5438, -72.939) (-67.6874, -72.4859) (-67.8308, -72.0327) knots 0 0 0 0 1 1 1 1
  spline S245 degree 3 poles (-67.8308, -72.0327) (-67.8993, -71.8166) (-67.9678, -71.6006) (-68.0365, -71.3847) knots 0 0 0 0 1 1 1 1
  spline S246 degree 3 poles (-68.0365, -71.3847) (-68.1322, -71.0833) (-68.2273, -70.7817) (-68.3224, -70.4801) knots 0 0 0 0 1 1 1 1
  spline S247 degree 3 poles (-68.3224, -70.4801) (-68.4036, -70.2234) (-68.4036, -70.2234) (-68.4865, -69.9615) knots 0 0 0 0 1 1 1 1
  spline S248 degree 3 poles (-68.4865, -69.9615) (-68.6083, -69.5435) (-68.7032, -69.1315) (-68.7806, -68.7033) knots 0 0 0 0 1 1 1 1
  spline S249 degree 3 poles (-68.7806, -68.7033) (-68.3615, -68.7033) (-67.9424, -68.7033) (-67.5106, -68.7033) knots 0 0 0 0 1 1 1 1
  spline S250 degree 3 poles (-67.5106, -68.7033) (-67.3243, -69.2751) (-67.1395, -69.8474) (-66.955, -70.4198) knots 0 0 0 0 1 1 1 1
  spline S251 degree 3 poles (-66.955, -70.4198) (-66.902, -70.5824) (-66.849, -70.745) (-66.7944, -70.9125) knots 0 0 0 0 1 1 1 1
  spline S252 degree 3 poles (-66.7944, -70.9125) (-66.7442, -71.0685) (-66.6941, -71.2246) (-66.6424, -71.3853) knots 0 0 0 0 1 1 1 1
  spline S253 degree 3 poles (-66.6424, -71.3853) (-66.5959, -71.5291) (-66.5493, -71.673) (-66.5013, -71.8211) knots 0 0 0 0 1 1 1 1
  spline S254 degree 3 poles (-66.5013, -71.8211) (-66.3993, -72.1958) (-66.3993, -72.1958) (-66.3993, -72.6721) knots 0 0 0 0 1 1 1 1
  spline S255 degree 3 poles (-66.3993, -72.6721) (-64.7753, -72.6721) (-63.1513, -72.6721) (-61.4781, -72.6721) knots 0 0 0 0 1 1 1 1
  spline S256 degree 3 poles (-61.4781, -72.6721) (-61.3733, -72.2006) (-61.2685, -71.7291) (-61.1606, -71.2433) knots 0 0 0 0 1 1 1 1
  spline S257 degree 3 poles (-61.1606, -71.2433) (-61.0265, -70.7877) (-60.8895, -70.3358) (-60.7439, -69.884) knots 0 0 0 0 1 1 1 1
  spline S258 degree 3 poles (-60.7439, -69.884) (-60.7074, -69.7693) (-60.671, -69.6546) (-60.6335, -69.5364) knots 0 0 0 0 1 1 1 1
  spline S259 degree 3 poles (-60.6335, -69.5364) (-60.5452, -69.2586) (-60.4561, -68.9809) (-60.3668, -68.7033) knots 0 0 0 0 1 1 1 1
  spline S260 degree 3 poles (-60.3668, -68.7033) (-59.9477, -68.7033) (-59.5286, -68.7033) (-59.0968, -68.7033) knots 0 0 0 0 1 1 1 1
  spline S261 degree 3 poles (-59.0968, -68.7033) (-59.8054, -71.1137) (-60.5627, -73.5074) (-61.3333, -75.8986) knots 0 0 0 0 1 1 1 1
  spline S262 degree 3 poles (-61.3333, -75.8986) (-61.4977, -76.4088) (-61.6617, -76.9191) (-61.8254, -77.4294) knots 0 0 0 0 1 1 1 1
  spline S263 degree 3 poles (-61.8254, -77.4294) (-61.9833, -77.9211) (-62.1415, -78.4127) (-62.2997, -78.9042) knots 0 0 0 0 1 1 1 1
  spline S264 degree 3 poles (-62.2997, -78.9042) (-62.3878, -79.1785) (-62.3878, -79.1785) (-62.4776, -79.4584) knots 0 0 0 0 1 1 1 1
  spline S265 degree 3 poles (-62.4776, -79.4584) (-62.5588, -79.7099) (-62.5588, -79.7099) (-62.6416, -79.9666) knots 0 0 0 0 1 1 1 1
  spline S266 degree 3 poles (-62.6416, -79.9666) (-62.6892, -80.1142) (-62.7367, -80.2619) (-62.7857, -80.414) knots 0 0 0 0 1 1 1 1
  spline S267 degree 3 poles (-62.7857, -80.414) (-62.9068, -80.7683) (-62.9068, -80.7683) (-63.0656, -81.0858) knots 0 0 0 0 1 1 1 1
  spline S268 degree 3 poles (-63.8593, -80.2921) (-63.1783, -78.0918) (-62.4973, -75.8915) (-61.7956, -73.6246) knots 0 0 0 0 1 1 1 1
  spline S269 degree 3 poles (-61.7956, -73.6246) (-63.2101, -73.6246) (-64.6245, -73.6246) (-66.0818, -73.6246) knots 0 0 0 0 1 1 1 1
  spline S270 degree 3 poles (-66.0818, -73.6246) (-65.806, -74.6359) (-65.5346, -75.6245) (-65.2118, -76.6179) knots 0 0 0 0 1 1 1 1
  spline S271 degree 3 poles (-65.2118, -76.6179) (-65.16, -76.778) (-65.16, -76.778) (-65.1071, -76.9414) knots 0 0 0 0 1 1 1 1
  spline S272 degree 3 poles (-65.1071, -76.9414) (-64.9991, -77.2746) (-64.8906, -77.6076) (-64.7821, -77.9406) knots 0 0 0 0 1 1 1 1
  spline S273 degree 3 poles (-64.7821, -77.9406) (-64.7077, -78.1697) (-64.6334, -78.3988) (-64.5591, -78.628) knots 0 0 0 0 1 1 1 1
  spline S274 degree 3 poles (-64.5591, -78.628) (-64.3792, -79.1828) (-64.1988, -79.7375) (-64.0181, -80.2921) knots 0 0 0 0 1 1 1 1
  spline S275 degree 3 poles (-64.0181, -80.2921) (-63.9657, -80.2921) (-63.9133, -80.2921) (-63.8593, -80.2921) knots 0 0 0 0 1 1 1 1
  spline S276 degree 3 poles (-116.7925, -77.8017) (-116.9953, -77.8043) (-117.1981, -77.807) (-117.4071, -77.8097) knots 0 0 0 0 1 1 1 1
  spline S277 degree 3 poles (-117.4071, -77.8097) (-118.0353, -77.7479) (-118.4121, -77.6073) (-118.9456, -77.2758) knots 0 0 0 0 1 1 1 1
  spline S278 degree 3 poles (-118.9456, -77.2758) (-119.7952, -76.2196) (-119.7621, -75.2537) (-119.7548, -73.9588) knots 0 0 0 0 1 1 1 1
  spline S279 degree 3 poles (-119.7548, -73.9588) (-119.7546, -73.8084) (-119.7544, -73.658) (-119.7542, -73.5031) knots 0 0 0 0 1 1 1 1
  spline S280 degree 3 poles (-119.7542, -73.5031) (-119.7533, -73.0243) (-119.7513, -72.5456) (-119.7493, -72.0668) knots 0 0 0 0 1 1 1 1
  spline S281 degree 3 poles (-119.7493, -72.0668) (-119.7485, -71.7416) (-119.7477, -71.4163) (-119.7471, -71.0911) knots 0 0 0 0 1 1 1 1
  spline S282 degree 3 poles (-119.7471, -71.0911) (-119.7453, -70.2952) (-119.7426, -69.4992) (-119.7393, -68.7033) knots 0 0 0 0 1 1 1 1
  spline S283 degree 3 poles (-119.7393, -68.7033) (-119.425, -68.7033) (-119.1107, -68.7033) (-118.7868, -68.7033) knots 0 0 0 0 1 1 1 1
  spline S284 degree 3 poles (-118.7868, -68.7033) (-118.7345, -68.9653) (-118.6821, -69.2272) (-118.6281, -69.4971) knots 0 0 0 0 1 1 1 1
  spline S285 degree 3 poles (-118.6281, -69.4971) (-118.5241, -69.4301) (-118.4202, -69.3632) (-118.3131, -69.2943) knots 0 0 0 0 1 1 1 1
  spline S286 degree 3 poles (-118.3131, -69.2943) (-117.112, -68.5733) (-116.0049, -68.1929) (-114.5967, -68.4571) knots 0 0 0 0 1 1 1 1
  spline S287 degree 3 poles (-114.5967, -68.4571) (-113.8789, -68.6875) (-113.4609, -69.0177) (-113.0718, -69.6558) knots 0 0 0 0 1 1 1 1
  spline S288 degree 3 poles (-113.0718, -69.6558) (-112.768, -70.4153) (-112.8543, -71.2126) (-113.0917, -71.9775) knots 0 0 0 0 1 1 1 1
  spline S289 degree 3 poles (-113.0917, -71.9775) (-113.7353, -73.136) (-114.7077, -73.5611) (-115.9293, -73.9421) knots 0 0 0 0 1 1 1 1
  spline S290 degree 3 poles (-115.9293, -73.9421) (-116.8231, -74.1787) (-117.7249, -74.3801) (-118.6281, -74.5771) knots 0 0 0 0 1 1 1 1
  spline S291 degree 3 poles (-118.6281, -74.5771) (-118.6389, -75.3366) (-118.6421, -75.9446) (-118.3106, -76.6408) knots 0 0 0 0 1 1 1 1
  spline S292 degree 3 poles (-118.3106, -76.6408) (-117.5227, -76.9376) (-116.5949, -76.8793) (-115.7706, -76.7996) knots 0 0 0 0 1 1 1 1
  spline S293 degree 3 poles (-115.7706, -76.7996) (-115.2269, -76.5563) (-115.2269, -76.5563) (-114.8181, -76.1646) knots 0 0 0 0 1 1 1 1
  spline S294 degree 3 poles (-114.8181, -76.1646) (-114.6397, -76.0188) (-114.4611, -75.8733) (-114.2823, -75.728) knots 0 0 0 0 1 1 1 1
  spline S295 degree 3 poles (-114.2823, -75.728) (-114.076, -75.5512) (-114.076, -75.5512) (-113.8656, -75.3708) knots 0 0 0 0 1 1 1 1
  spline S296 degree 3 poles (-113.8656, -75.3708) (-113.7084, -75.4756) (-113.5513, -75.5804) (-113.3893, -75.6883) knots 0 0 0 0 1 1 1 1
  spline S297 degree 3 poles (-113.3893, -75.6883) (-113.6071, -76.5111) (-114.1361, -76.9685) (-114.8181, -77.4346) knots 0 0 0 0 1 1 1 1
  spline S298 degree 3 poles (-114.8181, -77.4346) (-115.4797, -77.7722) (-116.0547, -77.7994) (-116.7925, -77.8017) knots 0 0 0 0 1 1 1 1
  spline S299 degree 3 poles (-114.5006, -72.1958) (-114.0202, -71.7154) (-113.8927, -71.2863) (-113.8656, -70.6083) knots 0 0 0 0 1 1 1 1
  spline S300 degree 3 poles (-113.8656, -70.6083) (-114.0687, -69.9989) (-114.2463, -69.7247) (-114.7685, -69.3482) knots 0 0 0 0 1 1 1 1
  spline S301 degree 3 poles (-114.7685, -69.3482) (-115.677, -69.0568) (-116.3936, -69.2296) (-117.2291, -69.626) knots 0 0 0 0 1 1 1 1
  spline S302 degree 3 poles (-117.2291, -69.626) (-117.5313, -69.7766) (-117.5313, -69.7766) (-117.8343, -69.9733) knots 0 0 0 0 1 1 1 1
  spline S303 degree 3 poles (-117.8343, -69.9733) (-117.9768, -70.0517) (-118.1192, -70.1301) (-118.2659, -70.2108) knots 0 0 0 0 1 1 1 1
  spline S304 degree 3 poles (-118.2659, -70.2108) (-118.8277, -70.8274) (-118.7142, -71.4333) (-118.6777, -72.2355) knots 0 0 0 0 1 1 1 1
  spline S305 degree 3 poles (-118.6777, -72.2355) (-118.6741, -72.3841) (-118.6705, -72.5326) (-118.6668, -72.6857) knots 0 0 0 0 1 1 1 1
  spline S306 degree 3 poles (-118.6668, -72.6857) (-118.6575, -73.0518) (-118.6445, -73.4174) (-118.6281, -73.7833) knots 0 0 0 0 1 1 1 1
  spline S307 degree 3 poles (-118.6281, -73.7833) (-117.3004, -73.7833) (-115.5196, -72.9907) (-114.5006, -72.1958) knots 0 0 0 0 1 1 1 1
  spline S308 degree 3 poles (-92.1863, -77.5239) (-93.0867, -76.9851) (-93.6408, -76.0358) (-93.9226, -75.0434) knots 0 0 0 0 1 1 1 1
  spline S309 degree 3 poles (-93.9226, -75.0434) (-94.0218, -74.4183) (-94.0218, -74.4183) (-94.0218, -73.1483) knots 0 0 0 0 1 1 1 1
  spline S310 degree 3 poles (-94.0218, -73.1483) (-91.9263, -73.1483) (-89.8308, -73.1483) (-87.6718, -73.1483) knots 0 0 0 0 1 1 1 1
  spline S311 degree 3 poles (-87.6718, -73.1483) (-88.0012, -71.2369) (-88.0012, -71.2369) (-88.6243, -70.2908) knots 0 0 0 0 1 1 1 1
  spline S312 degree 3 poles (-88.6243, -70.2908) (-88.6243, -70.186) (-88.6243, -70.0813) (-88.6243, -69.9733) knots 0 0 0 0 1 1 1 1
  spline S313 degree 3 poles (-88.6243, -69.9733) (-89.6547, -69.4185) (-90.4958, -69.2155) (-91.6406, -69.4971) knots 0 0 0 0 1 1 1 1
  spline S314 degree 3 poles (-91.6406, -69.4971) (-92.4233, -69.8958) (-92.7933, -70.3487) (-93.2281, -71.0846) knots 0 0 0 0 1 1 1 1
  spline S315 degree 3 poles (-93.2281, -71.0846) (-93.49, -70.9798) (-93.752, -70.875) (-94.0218, -70.7671) knots 0 0 0 0 1 1 1 1
  spline S316 degree 3 poles (-94.0218, -70.7671) (-93.851, -69.8526) (-93.2323, -69.2506) (-92.4939, -68.7232) knots 0 0 0 0 1 1 1 1
  spline S317 degree 3 poles (-92.4939, -68.7232) (-91.1396, -68.2717) (-89.7685, -68.2406) (-88.4656, -68.8621) knots 0 0 0 0 1 1 1 1
  spline S318 degree 3 poles (-88.4656, -68.8621) (-88.0092, -69.2292) (-88.0092, -69.2292) (-87.6718, -69.6558) knots 0 0 0 0 1 1 1 1
  spline S319 degree 3 poles (-87.6718, -69.6558) (-87.5572, -69.7999) (-87.4426, -69.9439) (-87.3246, -70.0924) knots 0 0 0 0 1 1 1 1
  spline S320 degree 3 poles (-87.3246, -70.0924) (-86.5033, -71.5649) (-86.4791, -73.5046) (-86.8979, -75.1128) knots 0 0 0 0 1 1 1 1
  spline S321 degree 3 poles (-86.8979, -75.1128) (-87.2503, -76.1093) (-87.7953, -76.9598) (-88.7136, -77.5139) knots 0 0 0 0 1 1 1 1
  spline S322 degree 3 poles (-88.7136, -77.5139) (-89.7722, -77.9691) (-91.1233, -77.9666) (-92.1863, -77.5239) knots 0 0 0 0 1 1 1 1
  spline S323 degree 3 poles (-88.2672, -75.8967) (-87.8969, -75.2519) (-87.8969, -75.2519) (-87.6718, -73.9421) knots 0 0 0 0 1 1 1 1
  spline S324 degree 3 poles (-87.6718, -73.9421) (-89.453, -73.9421) (-91.2342, -73.9421) (-93.0693, -73.9421) knots 0 0 0 0 1 1 1 1
  spline S325 degree 3 poles (-93.0693, -73.9421) (-92.7171, -75.5469) (-92.7171, -75.5469) (-91.7001, -76.7003) knots 0 0 0 0 1 1 1 1
  spline S326 degree 3 poles (-91.7001, -76.7003) (-90.3538, -77.3486) (-89.2144, -77.0281) (-88.2672, -75.8967) knots 0 0 0 0 1 1 1 1
  spline S327 degree 3 poles (-104.5688, -77.5239) (-105.4692, -76.9851) (-106.0233, -76.0358) (-106.3051, -75.0434) knots 0 0 0 0 1 1 1 1
  spline S328 degree 3 poles (-106.3051, -75.0434) (-106.4043, -74.4183) (-106.4043, -74.4183) (-106.4043, -73.1483) knots 0 0 0 0 1 1 1 1
  spline S329 degree 3 poles (-106.4043, -73.1483) (-104.3088, -73.1483) (-102.2133, -73.1483) (-100.0543, -73.1483) knots 0 0 0 0 1 1 1 1
  spline S330 degree 3 poles (-100.0543, -73.1483) (-100.3631, -71.4228) (-100.3631, -71.4228) (-101.1656, -70.1321) knots 0 0 0 0 1 1 1 1
  spline S331 degree 3 poles (-101.1656, -70.1321) (-101.2376, -70.0404) (-101.3097, -69.9487) (-101.3839, -69.8543) knots 0 0 0 0 1 1 1 1
  spline S332 degree 3 poles (-101.3839, -69.8543) (-101.9789, -69.3965) (-102.578, -69.3065) (-103.3087, -69.3582) knots 0 0 0 0 1 1 1 1
  spline S333 degree 3 poles (-103.3087, -69.3582) (-104.0928, -69.4728) (-104.6739, -69.7476) (-105.1746, -70.3857) knots 0 0 0 0 1 1 1 1
  spline S334 degree 3 poles (-105.1746, -70.3857) (-105.3288, -70.6129) (-105.4709, -70.8482) (-105.6106, -71.0846) knots 0 0 0 0 1 1 1 1
  spline S335 degree 3 poles (-105.6106, -71.0846) (-105.8725, -70.9798) (-106.1345, -70.875) (-106.4043, -70.7671) knots 0 0 0 0 1 1 1 1
  spline S336 degree 3 poles (-106.4043, -70.7671) (-106.3808, -69.9901) (-105.9692, -69.6269) (-105.4494, -69.1083) knots 0 0 0 0 1 1 1 1
  spline S337 degree 3 poles (-105.4494, -69.1083) (-104.529, -68.389) (-103.3358, -68.343) (-102.208, -68.4081) knots 0 0 0 0 1 1 1 1
  spline S338 degree 3 poles (-102.208, -68.4081) (-101.2135, -68.5667) (-100.5372, -69.0481) (-99.8956, -69.8146) knots 0 0 0 0 1 1 1 1
  spline S339 degree 3 poles (-99.8956, -69.8146) (-99.0198, -71.2725) (-98.8732, -73.0011) (-99.2159, -74.6496) knots 0 0 0 0 1 1 1 1
  spline S340 degree 3 poles (-99.2159, -74.6496) (-99.574, -75.9129) (-99.9369, -76.7915) (-101.0862, -77.4941) knots 0 0 0 0 1 1 1 1
  spline S341 degree 3 poles (-101.0862, -77.4941) (-102.1451, -77.9714) (-103.4975, -77.9701) (-104.5688, -77.5239) knots 0 0 0 0 1 1 1 1
  spline S342 degree 3 poles (-100.8481, -76.1646) (-100.3515, -75.4272) (-100.2029, -74.8333) (-100.0543, -73.9421) knots 0 0 0 0 1 1 1 1
  spline S343 degree 3 poles (-100.0543, -73.9421) (-101.8355, -73.9421) (-103.6167, -73.9421) (-105.4518, -73.9421) knots 0 0 0 0 1 1 1 1
  spline S344 degree 3 poles (-105.4518, -73.9421) (-105.0996, -75.5469) (-105.0996, -75.5469) (-104.0826, -76.7003) knots 0 0 0 0 1 1 1 1
  spline S345 degree 3 poles (-104.0826, -76.7003) (-102.9128, -77.2636) (-101.7361, -77.1447) (-100.8481, -76.1646) knots 0 0 0 0 1 1 1 1
  spline S346 degree 3 poles (-140.3768, -62.9883) (-140.8093, -62.7221) (-141.1494, -62.4126) (-141.4881, -62.0358) knots 0 0 0 0 1 1 1 1
  spline S347 degree 3 poles (-141.4881, -62.0358) (-141.6387, -62.1635) (-141.7893, -62.2912) (-141.9445, -62.4228) knots 0 0 0 0 1 1 1 1
  spline S348 degree 3 poles (-141.9445, -62.4228) (-142.6479, -63.0191) (-143.1596, -63.0414) (-144.0746, -63.0342) knots 0 0 0 0 1 1 1 1
  spline S349 degree 3 poles (-144.0746, -63.0342) (-144.6492, -62.9728) (-144.9246, -62.789) (-145.2981, -62.3533) knots 0 0 0 0 1 1 1 1
  spline S350 degree 3 poles (-145.2981, -62.3533) (-145.5003, -61.7466) (-145.4764, -61.1775) (-145.4723, -60.5457) knots 0 0 0 0 1 1 1 1
  spline S351 degree 3 poles (-145.4723, -60.5457) (-145.4721, -60.416) (-145.4719, -60.2863) (-145.4717, -60.1526) knots 0 0 0 0 1 1 1 1
  spline S352 degree 3 poles (-145.4717, -60.1526) (-145.4708, -59.7386) (-145.4688, -59.3245) (-145.4668, -58.9104) knots 0 0 0 0 1 1 1 1
  spline S353 degree 3 poles (-145.4668, -58.9104) (-145.466, -58.6296) (-145.4652, -58.3488) (-145.4646, -58.068) knots 0 0 0 0 1 1 1 1
  spline S354 degree 3 poles (-145.4646, -58.068) (-145.4628, -57.3798) (-145.4601, -56.6915) (-145.4568, -56.0033) knots 0 0 0 0 1 1 1 1
  spline S355 degree 3 poles (-145.4568, -56.0033) (-145.1425, -56.0033) (-144.8282, -56.0033) (-144.5043, -56.0033) knots 0 0 0 0 1 1 1 1
  spline S356 degree 3 poles (-144.5043, -56.0033) (-144.452, -57.994) (-144.3996, -59.9848) (-144.3456, -62.0358) knots 0 0 0 0 1 1 1 1
  spline S357 degree 3 poles (-144.3456, -62.0358) (-143.1923, -62.2226) (-143.1923, -62.2226) (-142.2818, -61.7183) knots 0 0 0 0 1 1 1 1
  spline S358 degree 3 poles (-142.2818, -61.7183) (-141.7931, -61.3408) (-141.6599, -61.1645) (-141.5602, -60.5449) knots 0 0 0 0 1 1 1 1
  spline S359 degree 3 poles (-141.5602, -60.5449) (-141.5552, -60.2306) (-141.5552, -60.2306) (-141.5501, -59.9101) knots 0 0 0 0 1 1 1 1
  spline S360 degree 3 poles (-141.5501, -59.9101) (-141.5475, -59.7982) (-141.5449, -59.6863) (-141.5421, -59.5711) knots 0 0 0 0 1 1 1 1
  spline S361 degree 3 poles (-141.5421, -59.5711) (-141.5345, -59.2153) (-141.5311, -58.8595) (-141.5278, -58.5036) knots 0 0 0 0 1 1 1 1
  spline S362 degree 3 poles (-141.5278, -58.5036) (-141.5233, -58.2618) (-141.5186, -58.0199) (-141.5135, -57.7781) knots 0 0 0 0 1 1 1 1
  spline S363 degree 3 poles (-141.5135, -57.7781) (-141.5018, -57.1865) (-141.4939, -56.595) (-141.4881, -56.0033) knots 0 0 0 0 1 1 1 1
  spline S364 degree 3 poles (-141.4881, -56.0033) (-141.1738, -56.0033) (-140.8594, -56.0033) (-140.5356, -56.0033) knots 0 0 0 0 1 1 1 1
  spline S365 degree 3 poles (-140.5356, -56.0033) (-140.5341, -56.1739) (-140.5326, -56.3446) (-140.5311, -56.5204) knots 0 0 0 0 1 1 1 1
  spline S366 degree 3 poles (-140.5311, -56.5204) (-140.5248, -57.1533) (-140.5143, -57.786) (-140.5026, -58.4189) knots 0 0 0 0 1 1 1 1